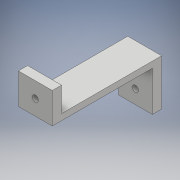
# Autodesk Inventor part: soporteOdroid
Saved by Autodesk Inventor 2017 (Build 210142000, 142)
## iProperties
Part Number: soporteOdroid
Material: Genérico
Document SubType Name: Modeling
Designer: Roberto
Density: 1 g/cm^3
Appearance: Valor por defecto
Author: Roberto
Autodesk Inventor part; units mm, degrees
ref_plane "YZ Plane" through (0, 0, 0) normal (1, 0, 0) x (0, 1, 0)
ref_plane "XZ Plane" through (0, 0, 0) normal (0, 1, 0) x (-1, 0, 0)
ref_plane "XY Plane" through (0, 0, 0) normal (0, 0, 1) x (1, 0, 0)
sketch "Boceto1" plane through (0, 0, 0) normal (0, 1, 0) x (-1, 0, 0)
  line L0 (0, 0) -> (0, 1)
  line L1 (0, 1) -> (1.1, 1)
  line L2 (1.1, 1) -> (1.1, 0)
  line L3 (1.1, 0) -> (0, 0)
  circle A0 centre (0.55, 0.5) radius 0.1
  dimension "d0" = 1
  dimension "d1" = 1.1
  dimension "d2" = 0.2
  constraints: 8 end point, 3 perpendicular, 1 centre point, 1 vertical
  measures "d0" distance of L0.start L0.end
  measures "d1" distance of L0.end L1.end
  measures "d2" diameter of A0
extrude "Extrusión1" add sketch "Boceto1" along normal blind 0.3
sketch "Boceto2" plane through (0, 0.3, 0) normal (0, 1, 0) x (1, 0, 0)
  line L0 (0, -1) -> (0, 0) projected
  line L1 (0, 0) -> (0, -0.2)
  line L2 (0, -0.2) -> (-1.1, -0.2)
  line L3 (-1.1, 0) -> (-1.1, -1) projected
  line L4 (-1.1, -0.2) -> (0, -0.2)
  line L5 (0, -0.2) -> (0, 0)
  line L6 (0, 0) -> (-1.1, 0)
  line L7 (-1.1, 0) -> (-1.1, -0.2)
  dimension "d5" = 0.2
  constraints: 12 end point, 2 parallel, 2 perpendicular, 2 point on line, 1 horizontal
  measures "d5" distance of L0.end L1.end
extrude "Extrusión2" add sketch "Boceto2" along normal blind 3.25
sketch "Boceto4" plane through (0, 3.55, 0) normal (0, 1, 0) x (1, 0, 0)
  circle A0 centre (-0.55, -0.5) radius 0.1 projected
  line L0 (0, 0) -> (-1.1, 0) projected
  line L1 (-1.1, 0) -> (-1.1, 1.3)
  line L2 (-1.1, 1.3) -> (0, 1.3)
  line L3 (0, 0) -> (0, -1) projected
  line L4 (0, 1.3) -> (0, 0)
  line L5 (0, 0) -> (-1.1, 0)
  circle A1 centre (-0.55, 0.85) radius 0.1
  dimension "d12" = 1.3
  dimension "d18" = 0.2
  constraints: 8 end point, 2 perpendicular, 1 centre point, 1 collinear, 1 vertical
  measures "d12" distance of L0.end L1.end
  measures "d18" diameter of A1
extrude "Extrusión4" add sketch "Boceto4" against normal blind 0.3 contours L0 L1 L2 L4
